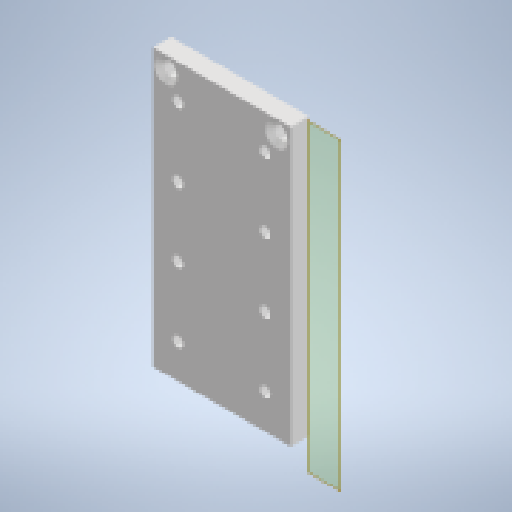
# Autodesk Inventor part: деталь которая двигает
Saved by Autodesk Inventor 2024.2 (Build 282272000, 272)
## iProperties
Created: 2025-11-27
Part Number: деталь которая двигает
Material: Типовые
Document SubType Name: Modeling
Designer: katya_notebook
Density: 1 g/cm^3
Appearance: По умолчанию
Author: katya_notebook
Autodesk Inventor part; units mm, degrees
ref_plane "YZ Plane" through (0, 0, 0) normal (1, 0, 0) x (0, 1, 0)
ref_plane "XZ Plane" through (0, 0, 0) normal (0, 1, 0) x (-1, 0, 0)
ref_plane "XY Plane" through (0, 0, 0) normal (0, 0, 1) x (1, 0, 0)
ref_plane "РабПлоскость2" through (101.7859, 42.6575, -2.4) normal (0, 0, -1) x (-1, 0, 0)
sketch "Эскиз2" plane through (101.7859, 42.6575, -2.4) normal (0, 0, -1) x (-1, 0, 0)
  line L0 (6.2, -87.5) -> (12.8, -87.5) projected
  line L1 (12.8, -27.5) -> (12.8, -87.5) projected
  line L2 (12.8, -27.5) -> (6.2, -27.5) projected
  line L3 (6.2, -27.5) -> (6.2, -87.5) projected
  circle A0 centre (9.5, -35) radius 2.3 projected
  circle A1 centre (9.5, -50) radius 2.3 projected
  circle A2 centre (9.5, -65) radius 2.3 projected
  circle A3 centre (9.5, -80) radius 2.3 projected
  line L4 (25.2, -87.5) -> (31.8, -87.5) projected
  line L5 (31.8, -27.5) -> (31.8, -87.5) projected
  line L6 (31.8, -27.5) -> (25.2, -27.5) projected
  line L7 (25.2, -27.5) -> (25.2, -87.5) projected
  circle A4 centre (28.5, -35) radius 2.3 projected
  circle A5 centre (28.5, -50) radius 2.3 projected
  circle A6 centre (28.5, -65) radius 2.3 projected
  circle A7 centre (28.5, -80) radius 2.3 projected
  line L8 (3.9216, -27.5) -> (33.9216, -27.5)
  line L9 (33.9216, -27.5) -> (33.9216, -87.5)
  line L10 (33.9216, -87.5) -> (3.9216, -87.5)
  line L11 (3.9216, -87.5) -> (3.9216, -27.5)
  line L12 (18.9216, -50) -> (18.9216, -69.7785)
  circle A8 centre (9.5, -35) radius 1.2 projected
  circle A9 centre (9.5, -50) radius 1.2 projected
  circle A10 centre (9.5, -65) radius 1.2 projected
  circle A11 centre (9.5, -80) radius 1.2 projected
  circle A12 centre (28.5, -80) radius 1.2 projected
  circle A13 centre (28.5, -65) radius 1.2 projected
  circle A14 centre (28.5, -50) radius 1.2 projected
  circle A15 centre (28.5, -35) radius 2.1 projected
  circle A16 centre (28.5, -35) radius 1.2 projected
  point P0 (101.7859, -42.6575)
  dimension "d3" = 30
  dimension "d4" = 60
  dimension "d5" = 15
  constraints: 10 end point, 2 parallel, 2 vertical, 1 horizontal, 1 perpendicular
  measures "d3" distance of L8.start L8.end
  measures "d4" distance of L8.end L9.end
  measures "d5" distance between parallel lines of L11 L12
extrude "Выдавливание2" add sketch "Эскиз2" along normal blind 4 contours L3 L2 L1 L0 | L10 L11 L8 L3 | L1 L8 L7 L10 | L7 L6 L5 L4 | L5 L8 L9 L10 | A0 | A1 | A2 | A3 | A4 | A5 | A6 | A7 | A15
sketch "Эскиз3" plane through (101.7859, 42.6575, -6.4) normal (0, 0, -1) x (-1, 0, 0)
  circle A0 centre (7, -34.5989) radius 2 projected
  circle A1 centre (31, -34.5989) radius 2 projected
  circle A2 centre (7, -30.55) radius 1.5 projected
  circle A3 centre (31, -30.55) radius 1.5 projected
  point P0 (101.7859, -42.6575)
extrude "Выдавливание3" cut sketch "Эскиз3" against normal blind 10 contours A2 | A3
chamfer "Фаска1" distance 1 angle 45 2 edges at (72.2859, 12.1075, -2.4) (96.2859, 12.1075, -2.4)
